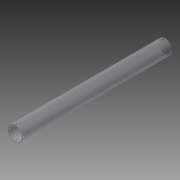
# Autodesk Inventor part: Polycarbonate Roller 2 OD 1-16 Thick (8585K64)
Saved by Autodesk Inventor 2014 (Build 180170000, 170)
## iProperties
Created: 2014-01-12
Part Number: Polycarbonate Roller 2 OD 1-16 Thick (8585K64)
Material: Polycarbonate, Clear
Document SubType Name: Modeling
Designer: Michael
Mass: 74.5407 g
Surface Area: 789.292 cm^2
Volume: 62.1173 cm^3
Density: 1.2 g/cm^3
Appearance: Polycarbonate - Clear
Author: Michael
Autodesk Inventor part; units mm, degrees
ref_plane "XY Plane" through (0, 0, 0) normal (0, 0, 1) x (1, 0, 0)
sketch "Sketch1" plane through (0, 0, 0) normal (0, 0, 1) x (1, 0, 0)
  circle A0 centre (0, 0) radius 25.4
  circle A1 centre (0, 0) radius 23.8125
  dimension "d0" = 50.8
  dimension "d1" = 47.625
  constraints: 2 centre point, 2 coincident
  measures "d0" diameter of A0
  measures "d1" diameter of A1
extrude "Extrusion1" add sketch "Sketch1" along normal blind 523.0622
ref_plane "Work Plane1" through (0, -25.4, 0) normal (0, 1, 0) x (-1, 0, 0)
sketch "Sketch2" plane through (0, -25.4, 0) normal (0, 1, 0) x (-1, 0, 0)
  line L0 (25.4, 523.0622) -> (-25.4, 523.0622) projected
  line L1 (-25.4, 0) -> (25.4, 0) projected
  line L2 (18.6459, 261.5311) -> (-13.1041, 261.5311) construction
  line L3 (25.4, 0) -> (25.4, 523.0622) construction
  line L4 (-25.4, 0) -> (-25.4, 523.0622) construction
  circle A0 centre (0, 5.5563) radius 2.413
  circle A1 centre (0, 517.5059) radius 2.413
  point P0 (0, 0)
  dimension "d4" = 261.5311
  dimension "d5" = 4.826
  dimension "d6" = 5.5563
  dimension "d7" = 25.4
  constraints: 2 centre point, 2 end point, 1 parallel, 1 symmetric about line, 1 other
  measures "d4" distance between parallel lines of L2 L1
  measures "d5" diameter of A0
  measures "d6" distance from line of L1 A0.centre
  measures "d7" distance from line of L3 A0.centre
extrude "Extrusion2" cut sketch "Sketch2" along normal blind 50.8
ref_plane "Work Plane2" through (25.4, 0, 0) normal (1, 0, 0) x (0, 1, 0)
sketch "Sketch3" plane through (25.4, 0, 0) normal (1, 0, 0) x (0, 1, 0)
  line L0 (-25.4, 0) -> (25.4, 0) projected
  line L1 (25.4, 0) -> (25.4, 523.0622) projected
  line L2 (-25.4, 0) -> (-25.4, 523.0622) projected
  line L3 (25.4, 523.0622) -> (-25.4, 523.0622) projected
  line L4 (25.4, 261.5311) -> (-25.4, 261.5311) construction
  circle A0 centre (0, 5.5563) radius 2.413
  circle A1 centre (0, 517.5059) radius 2.413
  point P0 (0, 0)
  dimension "d10" = 261.5311
  dimension "d11" = 4.826
  dimension "d12" = 5.5563
  dimension "d13" = 25.4
  constraints: 2 centre point, 2 end point, 2 midpoint, 1 perpendicular, 1 symmetric about line, 1 other
  measures "d10" distance between parallel lines of L3 L4
  measures "d11" diameter of A0
  measures "d12" distance from line of L0 A0.centre
  measures "d13" distance from line of A0.centre L2
extrude "Extrusion3" cut sketch "Sketch3" against normal blind 50.8 contours A0 | A1
equation "\"d4\" = 0.5 * d2"
equation "\"d7\" = 0.5 * d0"
equation "\"d10\" = 0.5 * d2"
equation "\"d13\" = 0.5 * d0"
equation "\"d2\" = 523.0622"
body "Solid1"
